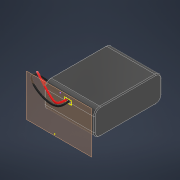
# Autodesk Inventor part: Batt_holder
Saved by Autodesk Inventor 2022 (Build 260153000, 153)
## iProperties
Created: 2022-03-27
Part Number: Batt_holder
Material: Generic
Document SubType Name: Modeling
Designer: dvorakj
Density: 1 g/cm^3
Appearance: Default
Author: dvorakj
Autodesk Inventor part; units mm, degrees
ref_plane "YZ Plane" through (0, 0, 0) normal (1, 0, 0) x (0, 1, 0)
ref_plane "XZ Plane" through (0, 0, 0) normal (0, 1, 0) x (-1, 0, 0)
ref_plane "XY Plane" through (0, 0, 0) normal (0, 0, 1) x (1, 0, 0)
sketch "Sketch1" plane through (0, 0, 0) normal (1, 0, 0) x (0, 1, 0)
  line L0 (0, 0) -> (30, 0)
  line L1 (30, 0) -> (30, -78)
  line L2 (30, -78) -> (0, -78)
  line L3 (0, -78) -> (0, 0)
  dimension "d0" = 30
  dimension "d1" = 78
  constraints: 8 end point, 2 parallel, 1 horizontal, 1 perpendicular
  measures "d0" distance of L1.end L2.end
  measures "d1" distance of L0.end L1.end
extrude "Extrusion1" add sketch "Sketch1" along normal mid plane 58
fillet "Fillet1" radius 7 4 edges at (0, 30, 0) (0, 0, 0) (0, 30, -78) (0, 0, -78)
fillet "Fillet2" radius 1 16 edges at (29, 27.9497, -2.0503) (29, 15, 0) (29, 2.0503, -2.0503) (29, 0, -39) (29, 2.0503, -75.9497) (29, 15, -78) (29, 27.9497, -75.9497) (29, 30, -39) (-29, 27.9497, -75.9497) (-29, 15, -78) (-29, 2.0503, -75.9497) (-29, 0, -39) (-29, 2.0503, -2.0503) (-29, 15, 0) (-29, 27.9497, -2.0503) (-29, 30, -39)
ref_plane "Work Plane1" through (10.618, 44.381, 16.9164) normal (-0.0022155, 0.0012275, 0.9999968) x (0.9999944, 0.0025158, 0.0022124)
sketch "Sketch3" plane through (10.618, 44.381, 16.9164) normal (-0.0022155, 0.0012275, 0.9999968) x (0.9999944, 0.0025158, 0.0022124)
  line L0 (8.353, -6.005) -> (0.663, -5.9857) projected
  line L1 (8.6538, -5.7058) -> (8.6645, -1.4358) projected
  line L2 (0.3745, -1.4149) -> (8.6645, -1.4358) projected
  line L3 (0.3745, -1.4149) -> (0.3638, -5.6849) projected
  line L4 (3.1483, -3.1619) -> (2.8083, -3.161) projected
  line L5 (3.1483, -3.1619) -> (3.1475, -3.5019) projected
  line L6 (5.8075, -3.5085) -> (5.8083, -3.1685) projected
  line L7 (6.1483, -3.1694) -> (5.8083, -3.1685) projected
  ellipse E0 centre (0.6638, -5.6857) end of major axis (0.5178, -5.9477) minor radius 0.3 (0.3638, -5.6849) -> (0.663, -5.9857) ccw projected
  ellipse E1 centre (8.3538, -5.705) end of major axis (8.4998, -5.443) minor radius 0.3 (8.353, -6.005) -> (8.6538, -5.7058) ccw projected
  point P0 (-10.767, -44.3333)
  point P1 (-3.9398, 0.1798)
  point P2 (2.9783, -3.3319)
  point P3 (5.9783, -3.3319)
  point P4 (3.1479, -3.3319)
  point P5 (2.9783, -3.1614)
  point P6 (5.9783, -3.169)
  constraints: 3 midpoint, 2 horizontal alignment, 2 vertical alignment, 2 other
sketch "Sketch5" plane through (-29, 0, 0) normal (-1, 0, 0) x (0, 0, 1)
  line L0 (0, 7) -> (0, 23) projected
  line L1 (-71, 0) -> (-7, 0) projected
  circle A0 centre (-18, 11) radius 1
  circle A1 centre (-14, 11) radius 1
  point P0 (0, 0)
  dimension "d20" = 18
  dimension "d21" = 11
  dimension "d22" = 2
  dimension "d23" = 2
  dimension "d24" = 2
  constraints: 2 centre point, 1 horizontal alignment
  measures "d20" distance from line of L0 A0.centre
  measures "d21" distance from line of L1 A0.centre
  measures "d22" diameter of A0
  measures "d23" diameter of A1
sketch3d "3D Sketch7"
  spline S0 degree 4 poles (-29, 11, -18) (-39.8021, 13.5089, -17.5987) (-40.8074, 34.2993, -2.4543) (-43.9024, 40.0707, 15.9796) (15.777, 34.8392, 32.0497) (16.6537, 40.9938, 23.9744) (16.6046, 41.0642, 16.9338) knots 1 1 1 1 1 2 3 4 4 4 4 4
sweep "Sweep4" add profiles "Sketch5" path "3D Sketch7" separate body contours A0
sketch3d "3D Sketch6"
  spline S0 degree 4 poles (-29, 11, -14) (-47.0193, 12.2076, -15.0813) (-49.2132, 41.2805, -4.2746) (-1.9169, 41.4447, 22.6978) (10.0834, 41.8794, 27.623) (13.6511, 41.7412, 27.7071) (13.6047, 41.0567, 16.9271) knots 1 1 1 1 1 2 3 4 4 4 4 4
sweep "Sweep5" add profiles "Sketch5" path "3D Sketch6" separate body contours A1
equation "\"d23\" = d22"
body "Solid1"
body "Solid2"
body "Solid3"
